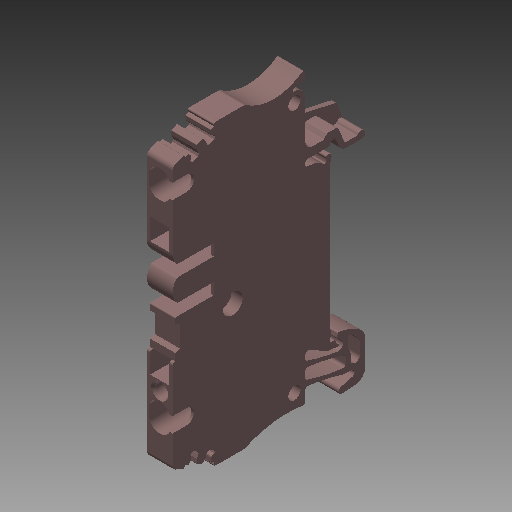
# Autodesk Inventor part: ZDU 2.5 1608510000
Saved by Autodesk Inventor 2019.3 (Build 233278000, 278)
## iProperties
Category: PARTsolutions
Company: WEIDMUELLER
Created: 2018-11-07
Part Number: ZDU 2.5 1608510000
Material: Generic
Catalog Web Link: www.cadenas.de
Description: ZDU 2.5-Feed-through terminals
Vendor: WEIDMUELLER
Document SubType Name: Modeling
Designer: psadmin
Manufacturer: WEIDMUELLER
Mass: 7.60708 g
Surface Area: 59.8519 cm^2
Volume: 7.60708 cm^3
Density: 1 g/cm^3
Appearance: PSOLRGB-175-140-135
PSOL_IDENT_0: {$CADENAS_DATA\23d-libs\weidmueller\reihenklemmen\z_series\durchgangs_rk\zdu2-5.prj},177 {VTYP=3D},{
PSOL_IDENT_1: NB=ZDU 2.5 1608510000},{LINA=ZDU 2.5 1608510000},{NN=ZDU 2.5},{DATE=31.03.2017 09:23:18},{GEOMDATE=0
PSOL_IDENT_2: 5.05.2015 08:49:00},{VERSION=},{LINEID=10},{WBVAR=},{WBNUMERIC=}  {NB=ZDU 2.5 1608510000},{LINA=ZDU
PSOL_IDENT_3: 2.5 1608510000},{KT=DUMMY},{BEST=1608510000},{BZ=ZDU 2.5},{M=Wemid},{F=beige},{FCODE=0.69,0.55,0.53,
PSOL_IDENT_4: 0.00}
NN: ZDU 2.5
NT: Feed-through terminals
NB: ZDU 2.5 1608510000
NBSYN: $BZ. $BEST.
LINA: ZDU 2.5 1608510000
BEST: 1608510000
BZ: ZDU 2.5
M: Wemid
F: beige
SUPPLIER: WEIDMUELLER
ARTICLENO: ZDU 2.5 1608510000
BOMINFO: ZDU 2.5 1608510000
CREATOR: CADENAS GmbH
Title: ZDU 2.5 1608510000
Author: Cadenas PARTsolutions
Comments: Feed-through terminals
Autodesk Inventor part; units mm, degrees
ref_plane "YZ Plane" through (0, 0, 0) normal (1, 0, 0) x (0, 1, 0)
ref_plane "XZ Plane" through (0, 0, 0) normal (0, 1, 0) x (-1, 0, 0)
ref_plane "XY Plane" through (0, 0, 0) normal (0, 0, 1) x (1, 0, 0)
sketch "Skizze_4" plane through (0, 0, 0) normal (1, 0, 0) x (0, 1, 0)
  line L0 (21.6468, 38.35) -> (4.3821, 38.35)
  arc A0 (4.3821, 38.35) -> (3.4582, 37.7327) centre (4.3821, 37.35) ccw
  line L1 (3.4582, 37.7327) -> (0.2511, 29.99)
  arc A1 (0.2511, 29.99) -> (0.175, 29.6074) centre (1.175, 29.6074) ccw
  line L2 (0.175, 29.6074) -> (0.175, 24.2573)
  arc A2 (0.175, 24.2573) -> (0.2652, 23.8422) centre (1.175, 24.2572) ccw
  arc A3 (2.0587, 16.2) -> (0.2652, 23.8422) centre (-17.9304, 15.5404) ccw
  arc A4 (1.8336, 12.4766) -> (2.0587, 16.2) centre (-17.9304, 15.5404) ccw
  arc A5 (1.8336, 12.4766) -> (2.3277, 11.9) centre (2.3277, 12.4) ccw
  line L3 (2.3277, 11.9) -> (4.2252, 11.9)
  arc A6 (4.7218, 11.3415) -> (4.2252, 11.9) centre (4.2252, 11.4) ccw
  arc A7 (3.2372, 4.5838) -> (4.7218, 11.3415) centre (-30.038, 15.4356) ccw
  arc A8 (1.3206, 4.635) -> (3.2372, 4.5838) centre (2.2865, 4.8938) ccw
  line L4 (1.3206, 4.635) -> (1.2761, 4.8008)
  arc A9 (1.2761, 4.8008) -> (-0.0003, 4.5898) centre (0.6483, 4.6326) ccw
  line L5 (-0.0003, 4.5898) -> (0.1793, 1.8682)
  arc A10 (0.1793, 1.8682) -> (2.175, 0) centre (2.175, 2) ccw
  line L6 (2.175, 0) -> (7.279, 0)
  arc A11 (7.279, 0) -> (9.3322, 1.0737) centre (7.279, 2.5) ccw
  arc A12 (9.3322, 1.0737) -> (10.8731, 4.774) centre (1.53, 6.4937) ccw
  arc A13 (10.8731, 4.774) -> (10.9287, 5.1695) centre (6.2508, 5.6248) ccw
  arc A14 (10.9287, 5.1695) -> (10.7445, 5.4352) centre (10.6798, 5.1937) ccw
  line L7 (10.7445, 5.4352) -> (10.1614, 5.5915)
  arc A15 (10.1614, 5.5915) -> (9.8467, 5.35) centre (10.0967, 5.35) ccw
  line L8 (9.8467, 5.35) -> (9.8467, 5.2)
  arc A16 (9.7698, 5.0424) -> (9.8467, 5.2) centre (9.6467, 5.2) ccw
  line L9 (9.7698, 5.0424) -> (8.9678, 4.4159)
  arc A17 (8.6663, 4.31) -> (8.9678, 4.4159) centre (8.66, 4.81) ccw
  arc A18 (7.6861, 5.4575) -> (8.6663, 4.31) centre (8.6751, 5.31) ccw
  arc A19 (9.1619, 11.5613) -> (7.6861, 5.4575) centre (42.3065, 0.3172) ccw
  arc A20 (9.6351, 11.9) -> (9.1619, 11.5613) centre (9.6351, 11.4) ccw
  line L10 (9.6351, 11.9) -> (10.3247, 11.9)
  arc A21 (10.8247, 11.4) -> (10.3247, 11.9) centre (10.3247, 11.4) ccw
  line L11 (10.8247, 11.4) -> (10.8247, 11.2303)
  arc A22 (10.7578, 10.9803) -> (10.8247, 11.2303) centre (10.3247, 11.2303) ccw
  line L12 (10.7578, 10.9803) -> (8.9508, 7.8506)
  arc A23 (8.9508, 7.8506) -> (8.7627, 7.297) centre (10.2498, 7.1006) ccw
  line L13 (8.7627, 7.297) -> (8.5024, 5.3262)
  arc A24 (8.5024, 5.3262) -> (8.7007, 5.1) centre (8.7007, 5.3) ccw
  line L14 (8.7007, 5.1) -> (8.7498, 5.1)
  arc A25 (8.7498, 5.1) -> (8.9498, 5.3) centre (8.7498, 5.3) ccw
  line L15 (8.9498, 5.3) -> (8.9498, 5.35)
  arc A26 (9.0829, 5.571) -> (8.9498, 5.35) centre (9.1998, 5.35) ccw
  line L16 (9.0829, 5.571) -> (9.8433, 5.9732)
  arc A27 (9.8433, 5.9732) -> (9.9498, 6.15) centre (9.7498, 6.15) ccw
  line L17 (9.9498, 6.15) -> (9.9498, 6.75)
  arc A28 (10.3275, 7.0398) -> (9.9498, 6.75) centre (10.2498, 6.75) ccw
  line L18 (10.3275, 7.0398) -> (11.3453, 6.767)
  arc A29 (11.3453, 6.767) -> (11.6042, 6.767) centre (11.4748, 7.25) ccw
  line L19 (11.6042, 6.767) -> (12.5966, 7.033)
  arc A30 (12.726, 7.05) -> (12.5966, 7.033) centre (12.7261, 6.55) ccw
  line L20 (12.726, 7.05) -> (40.3071, 7.05)
  arc A31 (40.566, 7.0159) -> (40.3071, 7.05) centre (40.3072, 6.05) ccw
  line L21 (40.566, 7.0159) -> (41.6925, 6.7141)
  arc A32 (41.6925, 6.7141) -> (42.2102, 6.7141) centre (41.9513, 7.68) ccw
  line L22 (42.2102, 6.7141) -> (42.3897, 6.7622)
  arc A33 (42.3897, 6.7622) -> (42.575, 7.0037) centre (42.325, 7.0037) ccw
  line L23 (42.575, 7.0037) -> (42.575, 7.526)
  arc A34 (42.575, 7.526) -> (42.2503, 7.7646) centre (42.325, 7.526) ccw
  arc A35 (41.6729, 7.7606) -> (42.2503, 7.7646) centre (41.955, 8.72) ccw
  line L24 (41.6729, 7.7606) -> (41.5045, 7.8101)
  arc A36 (41.3985, 8.2271) -> (41.5045, 7.8101) centre (41.575, 8.05) ccw
  arc A37 (41.3985, 8.2271) -> (42.575, 11.0604) centre (38.575, 11.0604) ccw
  line L25 (42.575, 11.0604) -> (42.575, 11.4)
  arc A38 (43.075, 11.9) -> (42.575, 11.4) centre (43.075, 11.4) ccw
  line L26 (43.075, 11.9) -> (43.375, 11.9)
  arc A39 (43.875, 11.4) -> (43.375, 11.9) centre (43.375, 11.4) ccw
  line L27 (43.875, 11.4) -> (43.875, 7.27)
  arc A40 (43.875, 7.27) -> (44.1092, 7.0205) centre (44.125, 7.27) ccw
  line L28 (44.1092, 7.0205) -> (44.4408, 6.9995)
  arc A41 (44.675, 6.75) -> (44.4408, 6.9995) centre (44.425, 6.75) ccw
  line L29 (44.675, 6.75) -> (44.675, 6)
  arc A42 (44.425, 5.75) -> (44.675, 6) centre (44.425, 6) ccw
  line L30 (44.425, 5.75) -> (44.33, 5.75)
  arc A43 (44.33, 5.75) -> (44.2344, 5.731) centre (44.3301, 5.5) ccw
  line L31 (44.2344, 5.731) -> (42.9627, 5.2042)
  arc A44 (42.9627, 5.2042) -> (41.975, 3.726) centre (43.575, 3.726) ccw
  line L32 (41.975, 3.726) -> (41.975, 0.5)
  arc A45 (41.975, 0.5) -> (42.646, 0.0301) centre (42.475, 0.5) ccw
  line L33 (42.646, 0.0301) -> (46.246, 1.3404)
  arc A46 (46.246, 1.3404) -> (46.5631, 1.7021) centre (46.075, 1.8103) ccw
  line L34 (46.5631, 1.7021) -> (48.5634, 10.7246)
  arc A47 (50.0279, 11.9) -> (48.5634, 10.7246) centre (50.0278, 10.4) ccw
  line L35 (50.0279, 11.9) -> (58.9724, 11.9)
  arc A48 (58.9724, 11.9) -> (59.378, 12.6923) centre (58.9724, 12.4) ccw
  arc A49 (58.4666, 14.25) -> (59.378, 12.6923) centre (67.0848, 18.2471) ccw
  arc A50 (59.295, 23.6849) -> (58.4666, 14.25) centre (67.0848, 18.2471) ccw
  arc A51 (59.295, 23.6849) -> (59.475, 24.2573) centre (58.475, 24.2572) ccw
  line L36 (59.475, 24.2573) -> (59.475, 29.6074)
  arc A52 (59.475, 29.6074) -> (59.3989, 29.99) centre (58.475, 29.6074) ccw
  line L37 (59.3989, 29.99) -> (56.1918, 37.7327)
  arc A53 (56.1918, 37.7327) -> (55.2679, 38.35) centre (55.2679, 37.35) ccw
  line L38 (55.2679, 38.35) -> (40.925, 38.35)
  arc A54 (40.925, 38.35) -> (38.885, 37.5496) centre (40.925, 35.35) ccw
  arc A55 (38.885, 37.5496) -> (38.725, 37.183) centre (39.225, 37.183) ccw
  line L39 (38.725, 37.183) -> (38.725, 30.15)
  line L40 (38.725, 30.15) -> (36.425, 30.15)
  line L41 (36.425, 30.15) -> (36.425, 37.183)
  arc A56 (36.425, 37.183) -> (36.265, 37.5496) centre (35.925, 37.183) ccw
  arc A57 (36.265, 37.5496) -> (32.185, 37.5496) centre (34.225, 35.35) ccw
  arc A58 (32.185, 37.5496) -> (32.025, 37.183) centre (32.525, 37.183) ccw
  line L42 (32.025, 37.183) -> (32.025, 30.15)
  line L43 (32.025, 30.15) -> (29.725, 30.15)
  line L44 (29.725, 30.15) -> (29.725, 37.55)
  arc A59 (29.725, 37.55) -> (29.475, 37.8) centre (29.475, 37.55) ccw
  line L45 (29.475, 37.8) -> (28.4482, 37.8)
  line L46 (28.4482, 37.8) -> (28.1882, 37)
  line L47 (28.1882, 37) -> (28.1882, 36.8)
  line L48 (28.1882, 36.8) -> (23.8382, 36.8)
  line L49 (23.8382, 36.8) -> (23.8382, 37)
  line L50 (23.8382, 37) -> (23.5783, 37.8)
  line L51 (23.5783, 37.8) -> (22.1443, 37.8)
  arc A60 (22.1443, 37.8) -> (21.6468, 38.35) centre (21.6468, 37.85) ccw
  constraints: 122 point on circle, 104 end point, 61 centre point
extrude "Extrusion1" add sketch "Skizze_4" along normal blind 5.1
sketch "Skizze_1" plane through (0, 0, 0) normal (1, 0, 0) x (0, 1, 0)
  line L0 (1.5215, 36.8461) -> (-1.4769, 29.6074)
  line L1 (-1.4769, 29.6074) -> (0.175, 29.6074)
  arc A0 (0.2511, 29.99) -> (0.175, 29.6074) centre (1.175, 29.6074) ccw
  line L2 (0.2511, 29.99) -> (0.2589, 30.0088)
  arc A1 (0.5855, 30.1441) -> (0.2589, 30.0088) centre (0.4899, 29.9131) ccw
  line L3 (0.5855, 30.1441) -> (0.8627, 30.0293)
  line L4 (0.8627, 30.0293) -> (1.1085, 30.6228)
  arc A2 (1.2088, 30.6842) -> (1.1085, 30.6228) centre (1.2009, 30.5845) ccw
  line L5 (1.2088, 30.6842) -> (1.9749, 30.6239)
  line L6 (1.9749, 30.6239) -> (2.1597, 30.5474)
  line L7 (2.1597, 30.5474) -> (2.3897, 29.9921)
  line L8 (2.3897, 29.9921) -> (2.69, 29.8677)
  line L9 (2.69, 29.8677) -> (3.0819, 30.0301)
  line L10 (3.0819, 30.0301) -> (3.5029, 31.0464)
  line L11 (3.5029, 31.0464) -> (3.3405, 31.4383)
  line L12 (3.3405, 31.4383) -> (2.4628, 31.8019)
  line L13 (2.4628, 31.8019) -> (1.8785, 32.301)
  arc A3 (1.851, 32.4153) -> (1.8785, 32.301) centre (1.9434, 32.377) ccw
  line L14 (1.851, 32.4153) -> (2.2853, 33.4637)
  arc A4 (2.3855, 33.5252) -> (2.2853, 33.4637) centre (2.3777, 33.4255) ccw
  line L15 (2.3855, 33.5252) -> (3.1517, 33.4649)
  line L16 (3.1517, 33.4649) -> (4.0294, 33.1013)
  line L17 (4.0294, 33.1013) -> (4.4213, 33.2637)
  line L18 (4.4213, 33.2637) -> (4.8423, 34.2799)
  line L19 (4.8423, 34.2799) -> (4.6799, 34.6719)
  line L20 (4.6799, 34.6719) -> (4.3797, 34.7963)
  line L21 (4.3797, 34.7963) -> (3.8244, 34.5663)
  line L22 (3.8244, 34.5663) -> (3.6396, 34.6428)
  line L23 (3.6396, 34.6428) -> (3.0552, 35.1419)
  arc A5 (3.0278, 35.2562) -> (3.0552, 35.1419) centre (3.1202, 35.218) ccw
  line L24 (3.0278, 35.2562) -> (3.2736, 35.8497)
  line L25 (3.2736, 35.8497) -> (2.9964, 35.9645)
  arc A6 (2.8611, 36.2912) -> (2.9964, 35.9645) centre (3.0921, 36.1955) ccw
  line L26 (2.8611, 36.2912) -> (1.5215, 36.8461)
  constraints: 54 end point, 14 point on circle, 7 centre point
extrude "Extrusion2" cut sketch "Skizze_1" along normal blind 5.1
sketch "Skizze_3" plane through (0, 0, 0) normal (1, 0, 0) x (0, 1, 0)
  line L0 (58.1285, 36.8461) -> (56.7889, 36.2912)
  arc A0 (56.6536, 35.9646) -> (56.7889, 36.2912) centre (56.5579, 36.1955) ccw
  line L1 (56.6536, 35.9646) -> (56.3764, 35.8497)
  line L2 (56.3764, 35.8497) -> (56.6222, 35.2562)
  arc A1 (56.5948, 35.1419) -> (56.6222, 35.2562) centre (56.5298, 35.218) ccw
  line L3 (56.5948, 35.1419) -> (56.0104, 34.6428)
  line L4 (56.0104, 34.6428) -> (55.8256, 34.5663)
  line L5 (55.8256, 34.5663) -> (55.2703, 34.7963)
  line L6 (55.2703, 34.7963) -> (54.9701, 34.6719)
  line L7 (54.9701, 34.6719) -> (54.8077, 34.2799)
  line L8 (54.8077, 34.2799) -> (55.2287, 33.2637)
  line L9 (55.2287, 33.2637) -> (55.6206, 33.1013)
  line L10 (55.6206, 33.1013) -> (56.4983, 33.4649)
  line L11 (56.4983, 33.4649) -> (57.2645, 33.5252)
  arc A2 (57.3647, 33.4637) -> (57.2645, 33.5252) centre (57.2723, 33.4255) ccw
  line L12 (57.3647, 33.4637) -> (57.799, 32.4153)
  arc A3 (57.7715, 32.301) -> (57.799, 32.4153) centre (57.7066, 32.377) ccw
  line L13 (57.7715, 32.301) -> (57.1872, 31.8019)
  line L14 (57.1872, 31.8019) -> (56.3095, 31.4383)
  line L15 (56.3095, 31.4383) -> (56.1471, 31.0464)
  line L16 (56.1471, 31.0464) -> (56.5681, 30.0301)
  line L17 (56.5681, 30.0301) -> (56.96, 29.8677)
  line L18 (56.96, 29.8677) -> (57.2603, 29.9921)
  line L19 (57.2603, 29.9921) -> (57.4903, 30.5474)
  line L20 (57.4903, 30.5474) -> (57.6751, 30.6239)
  line L21 (57.6751, 30.6239) -> (58.4412, 30.6842)
  arc A4 (58.5415, 30.6228) -> (58.4412, 30.6842) centre (58.4491, 30.5845) ccw
  line L22 (58.5415, 30.6228) -> (58.7873, 30.0293)
  line L23 (58.7873, 30.0293) -> (59.0642, 30.144)
  arc A5 (59.3882, 30.0149) -> (59.0642, 30.144) centre (59.1599, 29.913) ccw
  arc A6 (59.475, 29.6074) -> (59.3882, 30.0149) centre (58.475, 29.6074) ccw
  line L24 (59.475, 29.6074) -> (61.1269, 29.6074)
  line L25 (61.1269, 29.6074) -> (58.1285, 36.8461)
  constraints: 52 end point, 14 point on circle, 7 centre point
extrude "Extrusion3" cut sketch "Skizze_3" along normal blind 5.1
sketch "Skizze_5" plane through (0, 0, 0) normal (1, 0, 0) x (0, 1, 0)
  line L0 (7.505, 11.9) -> (6.3557, 11.9)
  arc A0 (6.3557, 11.9) -> (5.8825, 11.5616) centre (6.3557, 11.4) ccw
  arc A1 (5.8825, 11.5616) -> (4.2722, 4.4592) centre (39.0258, 0.3135) ccw
  arc A2 (4.2722, 4.4592) -> (4.7687, 3.9) centre (4.7687, 4.4) ccw
  line L1 (4.7687, 3.9) -> (5.9292, 3.9)
  arc A3 (5.9292, 3.9) -> (6.4029, 4.2401) centre (5.9292, 4.4) ccw
  arc A4 (6.4029, 4.2401) -> (8.0015, 11.3415) centre (-26.7582, 15.4356) ccw
  arc A5 (8.0015, 11.3415) -> (7.505, 11.9) centre (7.505, 11.4) ccw
  constraints: 12 point on circle, 6 centre point, 4 end point
extrude "Extrusion4" cut sketch "Skizze_5" along normal blind 5.1
sketch "Skizze_6" plane through (0.9, 0, 0) normal (1, 0, 0) x (0, 0, -1)
  arc A0 (-3.3264, 7.2636) -> (-3.2198, 6.955) centre (-2.8264, 7.2636) ccw
  arc A1 (-2.9, 6.0292) -> (-3.2198, 6.955) centre (-4.4, 6.0292) ccw
  line L0 (-2.9, 6.0292) -> (-2.9, 4.9194)
  arc A2 (-2.9, 4.9194) -> (-1, 4.9194) centre (-1.95, 4.9194) ccw
  line L1 (-1, 4.9194) -> (-1, 7.4228)
  arc A3 (-1, 7.4228) -> (-1.1516, 7.6526) centre (-1.25, 7.4228) ccw
  arc A4 (-1.5464, 8.2949) -> (-1.1516, 7.6526) centre (-0.8978, 8.2511) ccw
  arc A5 (-1.5464, 8.2949) -> (-1.6534, 8.5173) centre (-1.7958, 8.3118) ccw
  arc A6 (-1.6534, 8.5173) -> (-2.9728, 9.2666) centre (-6.4937, 1.53) ccw
  arc A7 (-2.9728, 9.2666) -> (-3.3264, 9.039) centre (-3.0764, 9.039) ccw
  line L2 (-3.3264, 9.039) -> (-3.3264, 7.2636)
  constraints: 16 point on circle, 8 centre point, 6 end point
extrude "Extrusion5" cut sketch "Skizze_6" along normal blind 5.1
sketch "Skizze_7" plane through (0.9, 0, 0) normal (1, 0, 0) x (0, 0, -1)
  arc A0 (-14.3007, 57.3489) -> (-14.1944, 56.8746) centre (-14.1903, 57.1246) ccw
  arc A1 (-12.4686, 56.1428) -> (-14.1944, 56.8746) centre (-14.2364, 54.375) ccw
  line L0 (-12.4686, 56.1428) -> (-12.0464, 55.7206)
  arc A2 (-11.9, 55.367) -> (-12.0464, 55.7206) centre (-12.4, 55.367) ccw
  line L1 (-11.9, 55.367) -> (-11.9, 47.075)
  arc A3 (-11.9, 47.075) -> (-10.4, 45.575) centre (-10.4, 47.075) ccw
  line L2 (-10.4, 45.575) -> (-8.5, 45.575)
  arc A4 (-8.5, 45.575) -> (-8.1428, 45.7251) centre (-8.5, 46.075) ccw
  line L3 (-8.1428, 45.7251) -> (-7.6531, 46.2249)
  arc A5 (-7.296, 46.375) -> (-7.6531, 46.2249) centre (-7.296, 45.875) ccw
  line L4 (-7.296, 46.375) -> (-5.7871, 46.375)
  arc A6 (-5.3252, 46.0664) -> (-5.7871, 46.375) centre (-5.7871, 45.875) ccw
  line L5 (-5.3252, 46.0664) -> (-4.1719, 43.2836)
  arc A7 (-4.1719, 43.2836) -> (-3.71, 42.975) centre (-3.71, 43.475) ccw
  line L6 (-3.71, 42.975) -> (-1.716, 42.975)
  arc A8 (-1.716, 42.975) -> (-1.4995, 43.1) centre (-1.716, 43.225) ccw
  arc A9 (-1.1065, 43.4298) -> (-1.4995, 43.1) centre (-0.85, 42.725) ccw
  line L7 (-1.1065, 43.4298) -> (-0.8778, 43.513)
  arc A10 (-0.2369, 43.2142) -> (-0.8778, 43.513) centre (-0.7068, 43.0432) ccw
  line L8 (-0.2369, 43.2142) -> (-0.0301, 42.646)
  line L9 (-0.0301, 42.646) -> (-0.0301, 58.9724)
  line L10 (-0.0301, 58.9724) -> (-11.9, 58.9724)
  line L11 (-11.9, 58.9724) -> (-11.9, 58.1061)
  arc A11 (-12.4, 57.6061) -> (-11.9, 58.1061) centre (-12.4, 58.1061) ccw
  line L12 (-12.4, 57.6061) -> (-13.1963, 57.6061)
  arc A12 (-13.1963, 57.6061) -> (-14.3007, 57.3489) centre (-13.1963, 55.1061) ccw
  constraints: 26 end point, 26 point on circle, 13 centre point
extrude "Extrusion6" cut sketch "Skizze_7" along normal blind 5.1
sketch "Skizze_8" plane through (0, 0, 38.35) normal (0, 0, 1) x (1, 0, 0)
  arc A0 (0.5, 10.15) -> (2.4, 8.725) centre (2.4526, 10.7743) ccw
  line L0 (2.4, 8.725) -> (2.7, 8.725)
  arc A1 (2.7, 8.725) -> (4.6, 10.15) centre (2.6474, 10.7743) ccw
  line L1 (4.6, 10.15) -> (4.6, 12.8)
  arc A2 (4.6, 12.8) -> (2.7, 14.225) centre (2.6474, 12.1757) ccw
  line L2 (2.7, 14.225) -> (2.4, 14.225)
  arc A3 (2.4, 14.225) -> (0.5, 12.8) centre (2.4526, 12.1757) ccw
  line L3 (0.5, 12.8) -> (0.5, 10.15)
  constraints: 8 end point, 8 point on circle, 4 centre point
extrude "Extrusion7" cut sketch "Skizze_8" against normal blind 8
sketch "Skizze_9" plane through (0, 0, 38.35) normal (0, 0, 1) x (1, 0, 0)
  arc A0 (0.5, 50.4) -> (2.4, 48.975) centre (2.4526, 51.0243) ccw
  line L0 (2.4, 48.975) -> (2.7, 48.975)
  arc A1 (2.7, 48.975) -> (4.6, 50.4) centre (2.6474, 51.0243) ccw
  line L1 (4.6, 50.4) -> (4.6, 53.05)
  arc A2 (4.6, 53.05) -> (2.7, 54.475) centre (2.6474, 52.4257) ccw
  line L2 (2.7, 54.475) -> (2.4, 54.475)
  arc A3 (2.4, 54.475) -> (0.5, 53.05) centre (2.4526, 52.4257) ccw
  line L3 (0.5, 53.05) -> (0.5, 50.4)
  constraints: 8 end point, 8 point on circle, 4 centre point
extrude "Extrusion8" cut sketch "Skizze_9" against normal blind 8
sketch "Skizze_10" plane through (5.1, 0, 0) normal (1, 0, 0) x (0, 0, -1)
  line L0 (-38.35, 12.975) -> (-38.35, 9.975)
  line L1 (-38.35, 9.975) -> (-35.59, 9.975)
  arc A0 (-35.59, 9.975) -> (-35.59, 12.975) centre (-35.59, 11.475) ccw
  line L2 (-35.59, 12.975) -> (-38.35, 12.975)
  constraints: 6 end point, 2 point on circle, 1 centre point
extrude "Extrusion9" cut sketch "Skizze_10" against normal blind 1
sketch "Skizze_11" plane through (5.1, 0, 0) normal (1, 0, 0) x (0, 0, -1)
  line L0 (-38.35, 53.225) -> (-38.35, 50.225)
  line L1 (-38.35, 50.225) -> (-35.59, 50.225)
  arc A0 (-35.59, 50.225) -> (-35.59, 53.225) centre (-35.59, 51.725) ccw
  line L2 (-35.59, 53.225) -> (-38.35, 53.225)
  constraints: 6 end point, 2 point on circle, 1 centre point
extrude "Extrusion10" cut sketch "Skizze_11" against normal blind 1
sketch "Sketch11" plane through (0, 4.3821, 38.35) normal (0, 0, 1) x (1, 0, 0)
  point P0 (2.55, 11.6929)
hole "Hole1" at (2.55, 16.075, 38.35) direction (0, 0, -1) diameter 2.8 depth 6 countersink diameter 3.3773 countersink angle 60
sketch "Skizze_13" plane through (2.55, 0, 0) normal (1, 0, 0) x (0, 0, -1)
  line L0 (-38.35, 17.925) -> (-30.35, 17.925)
  line L1 (-30.35, 17.925) -> (-30.35, 22.175)
  line L2 (-30.35, 22.175) -> (-38.35, 22.175)
  line L3 (-38.35, 22.175) -> (-38.35, 17.925)
  constraints: 8 end point
extrude "Extrusion11" cut sketch "Skizze_13" along normal mid plane 3.8
sketch "Skizze_14" plane through (2.55, 0, 0) normal (1, 0, 0) x (0, 0, -1)
  line L0 (-38.35, 40.925) -> (-30.35, 40.925)
  line L1 (-30.35, 40.925) -> (-30.35, 45.175)
  line L2 (-30.35, 45.175) -> (-38.35, 45.175)
  line L3 (-38.35, 45.175) -> (-38.35, 40.925)
  constraints: 8 end point
extrude "Extrusion12" cut sketch "Skizze_14" along normal mid plane 3.8
sketch "Sketch14" plane through (5.1, 0, 0) normal (1, 0, 0) x (0, 0, -1)
  point P0 (-14.05, 4.83)
hole "Hole2" at (5.1, 4.83, 14.05) direction (-1, 0, 0) diameter 2.5 depth 2.5
sketch "Sketch15" plane through (5.1, 0, 0) normal (1, 0, 0) x (0, 0, -1)
  point P0 (-14.05, 54.83)
hole "Hole3" at (5.1, 54.83, 14.05) direction (-1, 0, 0) diameter 2.5 depth 2.5
sketch "Sketch_3" plane through (0, 0, 30.15) normal (0, 0, 1) x (1, 0, 0)
  line L0 (0.9, 32.03) -> (0.9, 29.73)
  line L1 (0.9, 29.73) -> (4.6, 29.73)
  line L2 (4.6, 29.73) -> (4.6, 32.03)
  line L3 (4.6, 32.03) -> (0.9, 32.03)
  constraints: 8 end point
extrude "Extrusion13" cut sketch "Sketch_3" against normal blind 10
sketch "Sketch_4" plane through (0, 0, 30.15) normal (0, 0, 1) x (1, 0, 0)
  line L0 (0.9, 38.73) -> (0.9, 36.43)
  line L1 (0.9, 36.43) -> (4.6, 36.43)
  line L2 (4.6, 36.43) -> (4.6, 38.73)
  line L3 (4.6, 38.73) -> (0.9, 38.73)
  constraints: 8 end point
extrude "Extrusion14" cut sketch "Sketch_4" against normal blind 10
sketch "Sketch18" plane through (0, 0, 0) normal (-1, 0, 0) x (0, 0, 1)
  point P0 (14.05, 4.83)
hole "Hole4" at (0, 4.83, 14.05) direction (1, 0, 0) diameter 2.5 depth 2.5
sketch "Sketch19" plane through (0, 0, 0) normal (-1, 0, 0) x (0, 0, 1)
  point P0 (14.05, 54.83)
hole "Hole5" at (0, 54.83, 14.05) direction (1, 0, 0) diameter 2.5 depth 2.5
sketch "Sketch20" plane through (0, 0, 0) normal (-1, 0, 0) x (0, 0, 1)
  point P0 (26.35, 26.38)
hole "Hole6" at (0, 26.38, 26.35) direction (1, 0, 0) diameter 4 depth 2.2
sketch "Sketch21" plane through (5.1, 0, 0) normal (1, 0, 0) x (0, 0, -1)
  point P0 (-26.35, 26.38)
hole "Hole7" at (5.1, 26.38, 26.35) direction (-1, 0, 0) diameter 4 depth 2.2
sketch "Sketch_9" plane through (5.1, 0, 0) normal (1, 0, 0) x (0, 0, -1)
  line L0 (-4.635, 1.3206) -> (-2.5059, 1.891)
  arc A0 (-2.5059, 1.891) -> (-2.6612, 3.0706) centre (-2.6612, 2.4706) ccw
  line L1 (-2.6612, 3.0706) -> (-4.5838, 3.2372)
  arc A1 (-4.635, 1.3206) -> (-4.5838, 3.2372) centre (-4.8938, 2.2865) ccw
  constraints: 4 end point, 4 point on circle, 2 centre point
extrude "Extrusion15" cut sketch "Sketch_9" against normal blind 4.3
body "Solid1"
